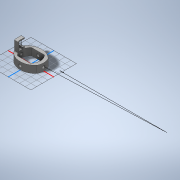
# Autodesk Inventor part: Part3
Saved by Autodesk Inventor 2022 (Build 260153000, 153)
## iProperties
Created: 2021-09-22
Part Number: Part3
Material: Generic
Document SubType Name: Modeling
Designer: WASHINGTON
Density: 1 g/cm^3
Appearance: Default
Author: WASHINGTON
Autodesk Inventor part; units mm, degrees
ref_plane "YZ Plane" through (0, 0, 0) normal (1, 0, 0) x (0, 1, 0)
ref_plane "XZ Plane" through (0, 0, 0) normal (0, 1, 0) x (-1, 0, 0)
ref_plane "XY Plane" through (0, 0, 0) normal (0, 0, 1) x (1, 0, 0)
sketch "Sketch1" plane through (0, 0, 0) normal (0, 1, 0) x (-1, 0, 0)
  line L0 (-22.2991, -25) -> (22.2991, -25)
  line L1 (22.2991, 25) -> (-22.2991, 25)
  arc A0 (-22.2991, 25) -> (-22.2991, -25) centre (0, 0) ccw
  arc A1 (22.2991, -25) -> (22.2991, 25) centre (0, 0) ccw
  line L2 (24.8747, 37.5) -> (-24.8747, 37.5)
  line L3 (24.8747, -37.5) -> (-24.8747, -37.5)
  arc A2 (24.8747, -37.5) -> (24.8747, 37.5) centre (0, 0) ccw
  arc A3 (-24.8747, 37.5) -> (-24.8747, -37.5) centre (0, 0) ccw
  circle A4 centre (0, 0) radius 25 construction
  arc A5 (0, 37.5) -> (-40.3994, 19.8214) centre (0, -17.5) ccw
  arc A6 (40.3994, 19.8214) -> (0, 37.5) centre (0, -17.5) ccw
  arc A7 (-40.3994, -19.8214) -> (0, -37.5) centre (0, 17.5) ccw
  arc A8 (0, -37.5) -> (40.3994, -19.8214) centre (0, 17.5) ccw
  point P0 (-40.0764, 20.168)
  point P1 (-40.0764, -20.168)
  point P2 (40.0764, 20.168)
  point P3 (40.0764, -20.168)
  dimension "d2" = 50
  dimension "d3" = 33.5
  dimension "d4" = 33.5
  dimension "d5" = 44.5982
  dimension "d7" = 12.5
  dimension "d8" = 12.5
  dimension "d54" = 45
  dimension "d55" = 45
  dimension "d60" = 55
  dimension "d61" = 55
  dimension "d62" = 55
  dimension "d63" = 55
  constraints: 24 point on circle, 9 centre point, 8 end point, 5 tangent, 3 coincident, 3 horizontal, 2 midpoint, 1 parallel
  measures "d2" distance between parallel lines of L0 L1
  measures "d3" radius of A0
  measures "d4" radius of A1
  measures "d5" distance of L0.start L0.end
  measures "d7" distance between parallel lines of L1 L2
  measures "d8" distance between parallel lines of L3 L0
  measures "d54" radius of A2
  measures "d55" radius of A3
  measures "d60" radius of A5
  measures "d61" radius of A6
  measures "d62" radius of A7
  measures "d63" radius of A8
extrude "Extrusion1" add sketch "Sketch1" along normal mid plane 25
sketch "Sketch3" plane through (0, 0, 0) normal (0, 0, 1) x (1, 0, 0)
  circle A0 centre (0, 0) radius 5
  dimension "d13" = 10
  constraints: 1 centre point, 1 coincident
  measures "d13" diameter of A0
extrude "Extrusion2" cut sketch "Sketch3" along normal through all both and the other way through all
sketch "Sketch5" plane through (0, 0, 0) normal (1, 0, 0) x (0, 1, 0)
  circle A0 centre (0, 0) radius 5
  dimension "d17" = 10
  constraints: 1 centre point, 1 coincident
  measures "d17" diameter of A0
extrude "Extrusion3" cut sketch "Sketch5" along normal through all both and the other way through all
sketch "Sketch6" plane through (0, 12.5, 0) normal (0, 1, 0) x (1, 0, 0)
  circle A0 centre (0, 0) radius 25 construction
  arc A1 (-22.2991, 25) -> (-22.2991, -25) centre (0, 0) ccw projected
  line L0 (-33.5, 0) -> (-47.5, 0) construction
  line L1 (-42.4264, -15) -> (-29.9541, -15)
  line L2 (-31.9726, 10) -> (-43.8748, 10)
  arc A2 (-24.8747, 37.5) -> (-24.8747, -37.5) centre (0, 0) ccw projected
  arc A3 (-43.8748, 10) -> (-43.9189, 9.8046) centre (0, 0) ccw
  line L3 (-32.5308, -8) -> (-44.2832, -8)
  arc A4 (-33.5, 0) -> (-29.9541, -15) centre (0, 0) ccw
  arc A5 (-43.9204, -9.798) -> (-42.4264, -15) centre (0, 0) ccw
  arc A6 (-43.8748, 10) -> (-43.9204, -9.798) centre (0, 0) ccw
  arc A7 (-31.9726, 10) -> (-33.5, 0) centre (0, 0) ccw
  line L4 (-44.7214, 5) -> (-33.1248, 5) projected
  arc A8 (-22.2991, 25) -> (-22.2991, -25) centre (0, 0) ccw projected
  line L5 (-33.2603, 4) -> (-44.8219, 4)
  point P0 (-44.2832, -8)
  point P1 (-44.8219, 4)
  dimension "d25" = 50
  dimension "d26" = 25
  dimension "d27" = 7
  dimension "d28" = 15
  dimension "d29" = 15
  dimension "d30" = 24.8046
  dimension "d31" = 5.202
  dimension "d32" = 47.5
  dimension "d37" = 6
  constraints: 21 point on circle, 10 end point, 6 centre point, 6 coincident, 3 parallel, 2 concentric, 2 horizontal, 2 other
  measures "d25" diameter of A0
  measures "d26" distance between parallel lines of L2 L1
  measures "d27" distance between parallel lines of L3 L1
  measures "d28" distance between parallel lines of L0 L1
  measures "d29" distance from line of point (0, 0) L1
  measures "d30" distance from line of A3.end L1
  measures "d31" distance from line of A5.start L1
  measures "d32" distance of A1.centre L0.end
  measures "d37" distance between parallel lines of L2 L5
extrude "Extrusion4" add sketch "Sketch6" along normal blind 6 contours A1 L4 A2 L2 | A1 L5 A2 L4 | A1 L3 A2 L5
extrude "Extrusion5" add sketch "Sketch6" along normal blind 33 contours A1 L1 A2 L3
extrude "Extrusion6" cut sketch "Sketch6" along normal through all contours A1 L3 A2 L5
sketch "Sketch7" plane through (-32.5308, 45.5, 8) normal (0, 0, -1) x (-1, 0, 0)
  line L0 (0, 0) -> (11.7524, 0) projected
  line L1 (-2.5766, -33) -> (-2.5766, 0) projected
  line L2 (11.7524, 0) -> (0, 0)
  line L3 (0, -3.5185) -> (15.3049, -3.5185)
  line L4 (15.3049, -3.5185) -> (11.7524, 0)
  line L5 (0, 0) -> (0, -3.5185)
  line L6 (0, -33) -> (0, 0) projected
  point P0 (-32.5308, -45.5)
  dimension "d40" = 5
  dimension "d41" = 15.3049
  constraints: 8 end point, 2 point on line, 1 horizontal, 1 parallel
  measures "d40" distance of L3.end L0.end
  measures "d41" distance of L3.start L3.end
extrude "Extrusion7" add sketch "Sketch7" along normal up to surface (18 mm away)
sketch "Sketch8" plane through (0, 45.5, 0) normal (0, 1, 0) x (1, 0, 0)
  circle A0 centre (0, 0) radius 45
  circle A1 centre (0, 0) radius 62.5
  dimension "d56" = 90
  dimension "d57" = 125
  constraints: 2 centre point, 2 coincident
  measures "d56" diameter of A0
  measures "d57" diameter of A1
extrude "Extrusion8" cut sketch "Sketch8" against normal through all
extrude "Extrusion9" cut sketch "Sketch1" along normal through all both and the other way through all contours A2 A6 L2 | A5 A3 L2 | A2 L3 A8 | A7 L3 A3
body "Solid1"
